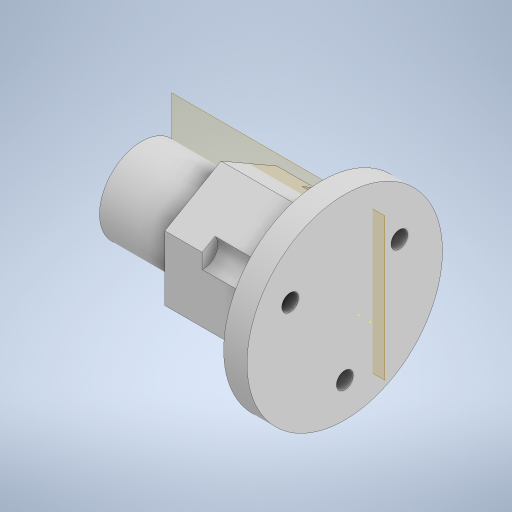
# Autodesk Inventor part: HEX HUB_Version2 (cheeta)
Saved by Autodesk Inventor 2024 (Build 280153000, 153)
## iProperties
Created: 2023-03-21
Part Number: HEX HUB_Version2 (cheeta)
Material: Generic
Document SubType Name: Modeling
Designer: Juyoung Han
Density: 1 g/cm^3
Appearance: Default
Mass: 7.90916 g
Surface Area: 51.3372 cm^2
Volume: 7.90916 cm^3
Author: Juyoung Han
Autodesk Inventor part; units mm, degrees
ref_plane "YZ Plane" through (0, 0, 0) normal (1, 0, 0) x (0, 1, 0)
ref_plane "XZ Plane" through (0, 0, 0) normal (0, 1, 0) x (-1, 0, 0)
ref_plane "XY Plane" through (0, 0, 0) normal (0, 0, 1) x (1, 0, 0)
sketch "Sketch1" plane through (0, 0, 0) normal (0, 0, 1) x (1, 0, 0)
  line L0 (0, 0) -> (-13, 0)
  line L1 (-13, 0) -> (-13, 9)
  line L2 (-13, 9) -> (0, 9)
  line L3 (0, 9) -> (0, 12)
  line L4 (0, 12) -> (8, 12)
  line L5 (8, 12) -> (8, 11)
  line L6 (33, 0) -> (0, 0)
  line L7 (8, 11) -> (8, 0)
  dimension "d0" = 13
  dimension "d1" = 9
  dimension "d2" = 13
  dimension "d3" = 3
  dimension "d4" = 8
  dimension "d5" = 1
  constraints: 16 end point, 5 perpendicular, 1 horizontal, 1 point on line, 1 vertical
  measures "d0" distance of L0.start L0.end
  measures "d1" distance of L0.end L1.end
  measures "d2" distance of L1.end L2.end
  measures "d3" distance of L2.end L3.end
  measures "d4" distance of L3.end L4.end
  measures "d5" distance of L4.end L5.end
sketch "Sketch1 outline for Revolution1" plane through (0, 0, 0) normal (0, 0, 1) x (1, 0, 0)
  line L0 (8, 11) -> (8, 12)
  line L1 (8, 0) -> (8, 11)
  line L2 (0, 0) -> (8, 0)
  line L3 (-13, 0) -> (0, 0)
  line L4 (-13, 9) -> (-13, 0)
  line L5 (0, 9) -> (-13, 9)
  line L6 (0, 12) -> (0, 9)
  line L7 (8, 12) -> (0, 12)
revolve "Revolution1" add sketch "Sketch1 outline for Revolution1" angle 360 about axis through (33, 0, 0) along (-1, 0, 0)
sketch "Sketch2" plane through (8, 0, 0) normal (1, 0, 0) x (0, 0, -1)
  circle A0 centre (0, 0) radius 12
  line L0 (12, -6.928203) -> (0, -13.856406)
  line L1 (0, -13.856406) -> (-12, -6.928203)
  line L2 (-12, -6.928203) -> (-12, 6.928203)
  line L3 (-12, 6.928203) -> (0, 13.856406)
  line L4 (0, 13.856406) -> (12, 6.928203)
  line L5 (12, 6.928203) -> (12, -6.928203)
  circle A1 centre (0, 0) radius 11
  point P0 (0, 0)
  point P1 (12, 0)
  point P2 (6, 10.392305)
  point P3 (6, -10.392305)
  point P4 (-6, 10.392305)
  point P5 (-12, 0)
  point P6 (-6, -10.392305)
  dimension "d12" = 24
  dimension "d13" = 0
  constraints: 12 end point, 2 coincident, 1 centre point, 13 other
  measures "d12" distance between parallel lines of L4 L1
  measures "d13" horizontal distance of point (0, 0) L3.end
sketch "Sketch2 outline for Extrusion1" plane through (8, 0, 0) normal (1, 0, 0) x (0, 0, -1)
  line L0 (12, 0) -> (12, 6.928203)
  arc A0 (6, 10.392305) -> (12, 0) centre (0, 0) cw
  line L1 (12, 6.928203) -> (6, 10.392305)
  line L2 (12, -6.928203) -> (12, 0)
  line L3 (6, -10.392305) -> (12, -6.928203)
  arc A1 (12, 0) -> (6, -10.392305) centre (0, 0) cw
  line L4 (6, 10.392305) -> (0, 13.856406)
  arc A2 (-6, 10.392305) -> (6, 10.392305) centre (0, 0) cw
  line L5 (0, 13.856406) -> (-6, 10.392305)
  line L6 (-6, 10.392305) -> (-12, 6.928203)
  arc A3 (-12, 0) -> (-6, 10.392305) centre (0, 0) cw
  line L7 (-12, 6.928203) -> (-12, 0)
  line L8 (-12, 0) -> (-12, -6.928203)
  arc A4 (-6, -10.392305) -> (-12, 0) centre (0, 0) cw
  line L9 (-12, -6.928203) -> (-6, -10.392305)
  line L10 (-6, -10.392305) -> (0, -13.856406)
  arc A5 (6, -10.392305) -> (-6, -10.392305) centre (0, 0) cw
  line L11 (0, -13.856406) -> (6, -10.392305)
extrude "Extrusion1" add sketch "Sketch2 outline for Extrusion1" against normal blind 8 contours A0 L1 L0 | L2 L3 A1 | A2 L5 L4 | L11 L10 A5 | A3 L7 L6 | L9 L8 A4
sketch "Sketch3" plane through (-13, 0, 0) normal (-1, 0, 0) x (0, 0, 1)
  circle A0 centre (0, 0) radius 7.75 projected
  circle A1 centre (0, 0) radius 6.5
  point P0 (0, 0)
  dimension "d18" = 13
  constraints: 1 centre point, 1 coincident
  measures "d18" diameter of A1
sketch "Sketch3 outline for Extrusion2" plane through (-13, 0, 0) normal (-1, 0, 0) x (0, 0, 1)
  circle A0 centre (0, 0) radius 6.5
extrude "Extrusion2" cut sketch "Sketch3 outline for Extrusion2" against normal blind 13
sketch "Sketch4" plane through (0, 0, 0) normal (-1, 0, 0) x (0, 0, 1)
  circle A0 centre (0, 0) radius 1.55
  point P0 (0, 0)
  dimension "d21" = 3.1
  constraints: 1 centre point, 1 coincident
  measures "d21" diameter of A0
sketch "Sketch4 outline for Extrusion3" plane through (0, 0, 0) normal (-1, 0, 0) x (0, 0, 1)
  circle A0 centre (0, 0) radius 1.55
extrude "Extrusion3" cut sketch "Sketch4 outline for Extrusion3" against normal through all
ref_plane "작업 평면2" through (20.5, 0, -6) normal (0, 0, 1) x (1, 0, 0)
sketch "스케치7" plane through (20.5, 0, -6) normal (0, 0, 1) x (1, 0, 0)
  circle A0 centre (6.75, 0) radius 1.3
  line L0 (6.75, -3.175426) -> (4, -1.587713)
  line L1 (4, -1.587713) -> (4, 1.587713)
  line L2 (4, 1.587713) -> (6.75, 3.175426)
  line L3 (6.75, 3.175426) -> (9.5, 1.587713)
  line L4 (9.5, 1.587713) -> (9.5, -1.587713)
  line L5 (9.5, -1.587713) -> (6.75, -3.175426)
  line L6 (12.5, 6) -> (12.5, -6)
  point P0 (-20.5, 0)
  point P1 (9.5, 0)
  dimension "d27" = 2.6
  dimension "d28" = 5.5
  dimension "d37" = 3
  constraints: 12 end point, 1 centre point, 1 coincident, 1 midpoint, 13 other
  measures "d27" diameter of A0
  measures "d28" distance from line of point (9.5, 0) L1
  measures "d37" distance between parallel lines of L6 L4
extrude "돌출6" [suppressed]
extrude "돌출7" [suppressed]
sketch "스케치8" plane through (33, 0, 0) normal (1, 0, 0) x (0, 0, -1)
  point P0 (0, 0)
sketch "스케치9" plane through (8, -6.928203, 12) normal (1, 0, 0) x (0, 0, -1)
  circle A0 centre (12, 6.928203) radius 16
  dimension "d38" = 32
  constraints: 1 centre point, 1 coincident
  measures "d38" diameter of A0
extrude "돌출8" [suppressed]
move faces "이동1" translate (12.5, 0, 10) faces at (8, 7.353412, -4.2935)
sketch "스케치10" plane through (20.5, -6.928203, 12) normal (1, 0, 0) x (0, 0, -1)
  circle A0 centre (12, 6.928203) radius 1.55
  circle A1 centre (12, 6.928203) radius 25
  dimension "d44" = 50
  constraints: 1 centre point, 1 coincident
  measures "d44" diameter of A1
extrude "돌출9" [suppressed]
sketch "스케치11" plane through (20.5, 0, 0) normal (-1, 0, 0) x (0, 0, 1)
  circle A0 centre (0, 0) radius 1.55 projected
  circle A1 centre (0, 0) radius 15
  circle A2 centre (0, 0) radius 16
  point P0 (0, 0)
  dimension "d49" = 30
  dimension "d50" = 32
  constraints: 2 centre point, 2 coincident
  measures "d49" diameter of A1
  measures "d50" diameter of A2
extrude "돌출10" [suppressed]
sketch "스케치12" plane through (20.5, -6.928203, 12) normal (1, 0, 0) x (0, 0, -1)
  circle A0 centre (12, 6.928203) radius 20.916385
  constraints: 1 centre point, 1 coincident
sketch "스케치12 outline for 돌출11" plane through (20.5, -6.928203, 12) normal (1, 0, 0) x (0, 0, -1)
  circle A0 centre (12, 6.928203) radius 20.916385
extrude "돌출11" add sketch "스케치12 outline for 돌출11" along normal blind 10
sketch "스케치14" plane through (30.5, 0, 0) normal (1, 0, 0) x (0, 0, -1)
  circle A0 centre (0, 0) radius 13.5
  circle A1 centre (0, -13.5) radius 1.795072
  circle A2 centre (11.691343, 6.75) radius 1.795072
  circle A3 centre (-11.691343, 6.75) radius 1.795072
  dimension "d59" = 27
  dimension "d64" = 360
  constraints: 3 centre point, 1 coincident, 1 vertical alignment, 9 other
sketch "스케치14 outline for 돌출13" plane through (30.5, 0, 0) normal (1, 0, 0) x (0, 0, -1)
  circle A0 centre (0, -13.5) radius 1.795072
  circle A1 centre (11.691343, 6.75) radius 1.795072
  circle A2 centre (-11.691343, 6.75) radius 1.795072
extrude "돌출13" cut sketch "스케치14 outline for 돌출13" against normal blind 15
sketch "스케치15" plane through (30.5, 0, 0) normal (1, 0, 0) x (0, 0, -1)
  point P0 (0, 0)
sketch "스케치16" plane through (20.5, 0, 0) normal (-1, 0, 0) x (0, 0, 1)
  circle A0 centre (0, -13.856406) radius 3
  circle A1 centre (11.691343, 6.75) radius 1.795072
  circle A2 centre (11.691343, 6.75) radius 3
  circle A3 centre (-12, 6.928203) radius 3
  point P0 (0, 0)
  dimension "d66" = 6
  dimension "d67" = 6
  dimension "d68" = 6
  constraints: 3 centre point, 1 coincident
  measures "d66" diameter of A3
  measures "d67" diameter of A2
  measures "d68" diameter of A0
sketch "스케치16 outline for 돌출14" plane through (20.5, 0, 0) normal (-1, 0, 0) x (0, 0, 1)
  circle A0 centre (11.691343, 6.75) radius 3
  circle A1 centre (-12, 6.928203) radius 3
  circle A2 centre (0, -13.856406) radius 3
extrude "돌출14" cut sketch "스케치16 outline for 돌출14" along normal blind 11.499
move faces "이동2" translate (-3, 0, 0) faces at (30.5, 0.037854, 0.072124)
move faces "이동3" translate (9, 0, 0) faces at (0, 0.36161, -10.978127)
move faces "이동4" translate (5, 0, 0) faces at (-13, 8.063695, 0.97911)
move faces "이동5" translate (-8, 0, 0) faces at (9, -0.36161, -10.978127)
move faces "이동6" translate (-25.75, 0, 0) faces at (13.666667, -0.124723, 1.544974)
move faces "이동7" translate (-8, 0, 0) faces at (-8, 8.063695, 0.97911)
move faces "이동8" translate (-36.5, 0, 0) faces at (20.5, -0.007186, -0.457486)
move faces "이동9" translate (-16, 0, 0) faces at (0, -0.518517, 4.787041)
move faces "이동10" translate (2, 0, 0) faces at (20.5, -1, -14.972128)
body "Solid1"
